mg400-gripper-attachment-v1 (Autodesk Fusion 360 design; units mm, degrees)
part number: 2026-10-04-11-29-29-067
Autodesk Fusion 360 part; units mm, degrees
sketch "Sketch1" plane through (0, 0, 0) normal (0, 0, 1) x (1, 0, 0)
  line L0 (-20, -55) -> (20, -55)
  line L1 (20, -55) -> (20, 55)
  line L2 (20, 55) -> (-20, 55)
  line L3 (-20, 55) -> (-20, -55)
  circle A0 centre (0, 0) radius 23
  circle A1 centre (0, 55) radius 20
  circle A2 centre (0, -55) radius 18
extrude "Extrude1" add sketch "Sketch1" along normal blind 5
sketch "Sketch2" plane through (0, 0, 0) normal (0, 0, 1) x (1, 0, 0)
  circle A0 centre (0, 0) radius 17
extrude "Extrude2" add sketch "Sketch2" along normal blind 14
ref_plane "WorkPlane2" through (0, 0, -38) normal (0, 0, 1) x (1, 0, 0)
sketch "Sketch4" plane through (0, 0, -38) normal (0, 0, 1) x (1, 0, 0)
  circle A0 centre (0, 55) radius 20
extrude "Extrude4" add sketch "Sketch4" along normal blind 46
ref_plane "WorkPlane3" through (0, 0, -6) normal (0, 0, 1) x (1, 0, 0)
sketch "Sketch5" plane through (0, 0, -6) normal (0, 0, 1) x (1, 0, 0)
  line L0 (-14.55, -8) -> (14.55, -8)
  line L1 (14.55, -8) -> (14.55, 8)
  line L2 (14.55, 8) -> (-14.55, 8)
  line L3 (-14.55, 8) -> (-14.55, -8)
extrude "Extrude5" add sketch "Sketch5" along normal blind 7
ref_plane "WorkPlane4" through (0, 0, -36) normal (0, 0, 1) x (1, 0, 0)
sketch "Sketch6" plane through (0, 0, -36) normal (0, 0, 1) x (1, 0, 0)
  line L0 (-12.15, -8) -> (-14.55, -8)
  line L1 (-14.55, -8) -> (-14.55, 8)
  line L2 (-14.55, 8) -> (-12.15, 8)
  line L3 (-12.15, 8) -> (-12.15, -8)
  line L4 (12.15, -8) -> (14.55, -8)
  line L5 (14.55, -8) -> (14.55, 8)
  line L6 (14.55, 8) -> (12.15, 8)
  line L7 (12.15, 8) -> (12.15, -8)
extrude "Extrude6" add sketch "Sketch6" along normal blind 31
ref_plane "WorkPlane5" through (0, 0, -36) normal (0, 0, 1) x (1, 0, 0)
sketch "Sketch7" plane through (0, 0, -36) normal (0, 0, 1) x (1, 0, 0)
  line L0 (-10.55, -8) -> (-14.55, -8)
  line L1 (-14.55, -8) -> (-14.55, 8)
  line L2 (-14.55, 8) -> (-10.55, 8)
  line L3 (-10.55, 8) -> (-10.55, -8)
  line L4 (10.55, -8) -> (14.55, -8)
  line L5 (14.55, -8) -> (14.55, 8)
  line L6 (14.55, 8) -> (10.55, 8)
  line L7 (10.55, 8) -> (10.55, -8)
extrude "Extrude7" add sketch "Sketch7" along normal blind 2.5
ref_plane "WorkPlane6" through (0, 0, -7) normal (0, 0, 1) x (1, 0, 0)
sketch "Sketch8" plane through (0, 0, -7) normal (0, 0, 1) x (1, 0, 0)
  circle A0 centre (8.4853, 8.4853) radius 1.7
  circle A1 centre (-8.4853, 8.4853) radius 1.7
  circle A2 centre (-8.4853, -8.4853) radius 1.7
  circle A3 centre (8.4853, -8.4853) radius 1.7
extrude "Extrude8" cut sketch "Sketch8" along normal blind 22
ref_plane "WorkPlane7" through (0, 0, -7) normal (0, 0, 1) x (1, 0, 0)
sketch "Sketch9" plane through (0, 0, -7) normal (0, 0, 1) x (1, 0, 0)
  circle A0 centre (0, 0) radius 6
extrude "Extrude9" cut sketch "Sketch9" along normal blind 22
ref_plane "WorkPlane8" through (0, 0, -21) normal (0, 0, 1) x (1, 0, 0)
sketch "Sketch10" plane through (0, 0, -21) normal (0, 0, 1) x (1, 0, 0)
  circle A0 centre (0, -55) radius 6
extrude "Extrude10" cut sketch "Sketch10" along normal blind 30
ref_plane "WorkPlane9" through (0, 0, -39) normal (0, 0, 1) x (1, 0, 0)
sketch "Sketch11" plane through (0, 0, -39) normal (0, 0, 1) x (1, 0, 0)
  circle A0 centre (0, 55) radius 8.4
extrude "Extrude11" cut sketch "Sketch11" along normal blind 48
ref_plane "WorkPlane10" through (0, 0, -3.5) normal (0, 0, 1) x (1, 0, 0)
sketch "Sketch12" plane through (0, 0, -3.5) normal (0, 0, 1) x (1, 0, 0)
  circle A0 centre (0, 55) radius 16
extrude "Extrude12" cut sketch "Sketch12" along normal blind 12.5
ref_plane "WorkPlane11" through (0, 0, -39) normal (0, 0, 1) x (1, 0, 0)
sketch "Sketch13" plane through (0, 0, -39) normal (0, 0, 1) x (1, 0, 0)
  line L0 (0, 54.4) -> (40, 54.4)
  line L1 (40, 54.4) -> (40, 55.6)
  line L2 (40, 55.6) -> (0, 55.6)
  line L3 (0, 55.6) -> (0, 54.4)
extrude "Extrude13" cut sketch "Sketch13" along normal blind 36.5
ref_plane "WorkPlane12" through (0, 55, 0) normal (0, 1, 0) x (0, 0, 1)
sketch "Sketch14" plane through (0, 55, 0) normal (0, 1, 0) x (1, 0, 0)
  circle A0 centre (14, 21) radius 1.6
extrude "Extrude14" cut sketch "Sketch14" along normal mid plane 50
sketch "CupBossHoles" plane through (0, 0, -21) normal (0, 0, 1) x (1, 0, 0)
  circle A0 centre (-8.5, -63.5) radius 1.7
  circle A1 centre (-8.5, -46.5) radius 1.7
  circle A2 centre (8.5, -63.5) radius 1.7
  circle A3 centre (8.5, -46.5) radius 1.7
extrude "CupBossHolesCut" cut sketch "CupBossHoles" along normal blind 30
sketch "CupScrewCounterbores" plane through (0, 0, 0) normal (0, 0, 1) x (1, 0, 0)
  circle A0 centre (-8.5, -63.5) radius 3.25
  circle A1 centre (-8.5, -46.5) radius 3.25
  circle A2 centre (8.5, -63.5) radius 3.25
  circle A3 centre (8.5, -46.5) radius 3.25
extrude "CupScrewCounterboresCut" cut sketch "CupScrewCounterbores" along normal through all from surface at 2
sketch "MainScrewCounterbores" plane through (0, 0, -7) normal (0, 0, 1) x (1, 0, 0)
  circle A0 centre (-8.5, -8.5) radius 3.25
  circle A1 centre (-8.5, 8.5) radius 3.25
  circle A2 centre (8.5, -8.5) radius 3.25
  circle A3 centre (8.5, 8.5) radius 3.25
extrude "MainScrewCounterboresCut" cut sketch "MainScrewCounterbores" along normal blind 19
